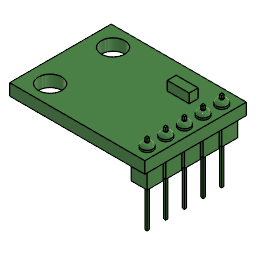
Dhanip_light-sensor (Autodesk Fusion 360 design; units mm, degrees)
Autodesk Fusion 360 part; units mm, degrees
note: some values were not read from the file. Set by a fixed rule: which sketch regions a step uses; which face or edge a step refers to.
sketch "Sketch1" plane through (0, 0, 0) normal (0, 0, 1) x (1, 0, 0)
sketch "Sketch2" plane through (0, 0, 0) normal (0, 0, 1) x (1, 0, 0)
  line L0 (9.25, -6.95) -> (-9.25, -6.95)
  line L1 (-9.25, -6.95) -> (-9.25, 6.95)
  line L2 (-9.25, 6.95) -> (9.25, 6.95)
  line L3 (9.25, 6.95) -> (9.25, -6.95)
  line L4 (9.25, -6.95) -> (-9.25, 6.95) construction
  line L5 (-9.25, -6.95) -> (9.25, 6.95) construction
  dimension "d3" = 18.5
  dimension "d4" = 13.9
  constraint horizontal L0
  constraint perpendicular L0 L1
  constraint parallel L0 L2
  constraint parallel L1 L3
  constraint coincident L4 origin
  constraint coincident L5 origin
  measures "d3" distance of L1.end L2.end
  measures "d4" distance of L0.end L1.end
extrude "Extrude1" add sketch "Sketch2" along normal blind 1.6
sketch "Sketch6" plane through (0, 0, 1.6) normal (0, 0, 1) x (-1, 0, 0)
  line L0 (-9.25, -6.95) -> (9.25, -6.95)
  line L1 (9.25, -6.95) -> (9.25, 6.95)
  line L2 (9.25, 6.95) -> (-9.25, 6.95)
  line L3 (-9.25, 6.95) -> (-9.25, -6.95)
  line L4 (9.25, 6.95) -> (6.35, 6.95)
  line L5 (9.25, 6.95) -> (9.25, 4.3)
  line L6 (9.25, 4.3) -> (5.4, 4.3)
  line L7 (6.35, 6.95) -> (6.35, 4.3)
  circle A0 centre (6.35, 4.3) radius 1.6
  dimension "d18" = 2.9
  dimension "d19" = 2.65
  dimension "d20" = 3.2
  constraint coincident L1.end L2.start
  constraint perpendicular L1 L4
  constraint perpendicular L2 L5
  constraint perpendicular L5 L6
  constraint coincident L6 L7.end
  constraint perpendicular L6 L7
  constraint coincident L7.end A0.centre
  measures "d18" distance of L1.end L4.end
  measures "d19" distance of L1.end L5.end
  measures "d20" diameter of A0
extrude "Extrude5" cut sketch "Sketch6" against normal blind 1.6 contours L6 L7 A0 | L6 L7 A0
mirror "Mirror2" about plane through (0, 0, 0) normal (0, 1, 0) of "Extrude5"
sketch "Sketch7" plane through (0, 0, 1.6) normal (0, 0, 1) x (-1, 0, 0)
  circle A0 centre (6.35, -4.3) radius 1.6
  circle A1 centre (6.35, 4.3) radius 1.6
  line L0 (-9.25, -6.95) -> (9.25, -6.95)
  line L1 (9.25, -6.95) -> (9.25, 6.95)
  line L2 (9.25, 6.95) -> (-9.25, 6.95)
  line L3 (-9.25, 6.95) -> (-9.25, -6.95)
  line L4 (-9.25, -4.9302) -> (-7.883, -4.9302)
  line L5 (-7.883, -4.9302) -> (-7.883, -6.95)
  line L6 (-7.883, -6.95) -> (-9.25, -6.95)
  line L7 (-7.883, -6.95) -> (-7.883, -4.926)
  circle A2 centre (-7.883, -4.9302) radius 0.7705
  dimension "d25" = 1.367
  dimension "d26" = 2.024
  dimension "d27" = 1.541
  constraint coincident L3 L4.start
  constraint perpendicular L3 L4
  constraint coincident L0 L5.end
  constraint perpendicular L0 L5
  constraint coincident L0.start L3.end
  constraint perpendicular L0 L7
  constraint coincident L4.end L5.start
  measures "d25" distance of L4.start L4.end
  measures "d26" distance of L5.end L7.end
  measures "d27" diameter of A2
extrude "Extrude6" add sketch "Sketch7" along normal blind 0.765 contours L4 L5 L7 A2 | L4 L5 L7 A2
sketch "Sketch8" plane through (0, 0, 2.365) normal (0, 0, 1) x (-1, 0, 0)
  circle A0 centre (-7.883, -4.9302) radius 0.7705
  line L0 (-7.733, -5.0802) -> (-8.033, -5.0802)
  line L1 (-8.033, -5.0802) -> (-8.033, -4.7802)
  line L2 (-8.033, -4.7802) -> (-7.733, -4.7802)
  line L3 (-7.733, -4.7802) -> (-7.733, -5.0802)
  line L4 (-7.733, -5.0802) -> (-8.033, -4.7802) construction
  line L5 (-8.033, -5.0802) -> (-7.733, -4.7802) construction
  point P0 (-7.883, -4.9302)
  dimension "d30" = 0.3
  dimension "d31" = 0.3
  constraint horizontal L0
  constraint perpendicular L0 L1
  constraint parallel L0 L2
  constraint parallel L1 L3
  constraint coincident L4 P0
  constraint coincident L5 P0
  constraint coincident P0 A0.centre
  measures "d30" distance of L1.end L2.end
  measures "d31" distance of L0.end L1.end
extrude "Extrude7" add sketch "Sketch8" along normal blind 0.531 contours L0 L1 L2 L3
fillet "Fillet1" radius 0.525 1 edges at (8.6014, 5.2088, 2.365)
pattern_linear "R-Pattern1" count 5 spacing 2.55 along (0, -1, 0) of "Extrude6", "Extrude7", "Fillet1"
extrude "Extrude8" add 5 faces at (7.833, 4.8802, 2.896) (7.833, 2.3302, 2.896) (7.833, -0.2198, 2.896) (7.833, -2.7698, 2.896) (7.833, -5.3198, 2.896) along direction (0, 0, -1) blind 11
sketch "Sketch9" plane through (0, 0, 0) normal (0, 0, -1) x (1, 0, 0)
  line L0 (8.033, 5.4198) -> (8.033, 5.1198)
  line L1 (8.033, 5.1198) -> (7.733, 5.1198)
  line L2 (7.733, 5.1198) -> (7.733, 5.4198)
  line L3 (7.733, 5.4198) -> (8.033, 5.4198)
  line L4 (8.033, 0.3198) -> (8.033, 0.0198)
  line L5 (8.033, 0.0198) -> (7.733, 0.0198)
  line L6 (7.733, 0.0198) -> (7.733, 0.3198)
  line L7 (7.733, 0.3198) -> (8.033, 0.3198)
  line L8 (8.033, -4.7802) -> (8.033, -5.0802)
  line L9 (8.033, -5.0802) -> (7.733, -5.0802)
  line L10 (7.733, -5.0802) -> (7.733, -4.7802)
  line L11 (7.733, -4.7802) -> (8.033, -4.7802)
  line L12 (8.033, -2.2302) -> (8.033, -2.5302)
  line L13 (8.033, -2.5302) -> (7.733, -2.5302)
  line L14 (7.733, -2.5302) -> (7.733, -2.2302)
  line L15 (7.733, -2.2302) -> (8.033, -2.2302)
  line L16 (8.033, 2.8698) -> (8.033, 2.5698)
  line L17 (8.033, 2.5698) -> (7.733, 2.5698)
  line L18 (7.733, 2.5698) -> (7.733, 2.8698)
  line L19 (7.733, 2.8698) -> (8.033, 2.8698)
  circle A0 centre (-6.35, -4.3) radius 1.6
  circle A1 centre (-6.35, 4.3) radius 1.6
  line L20 (-9.25, -6.95) -> (9.25, -6.95)
  line L21 (9.25, -6.95) -> (9.25, 6.95)
  line L22 (9.25, 6.95) -> (-9.25, 6.95)
  line L23 (-9.25, 6.95) -> (-9.25, -6.95)
  line L24 (7.733, 5.4198) -> (8.033, 5.1198)
  line L25 (7.733, 5.1198) -> (8.033, 5.4198)
  line L26 (8.983, 6.3698) -> (6.783, 6.3698)
  line L27 (6.783, 6.3698) -> (6.783, 4.1698)
  line L28 (6.783, 4.1698) -> (8.983, 4.1698)
  line L29 (8.983, 4.1698) -> (8.983, 6.3698)
  line L30 (8.983, 6.3698) -> (6.783, 4.1698) construction
  line L31 (6.783, 6.3698) -> (8.983, 4.1698) construction
  line L32 (7.733, 2.8698) -> (8.033, 2.5698)
  line L33 (8.033, 2.8698) -> (7.733, 2.5698)
  line L34 (8.983, 1.6198) -> (6.783, 1.6198)
  line L35 (6.783, 1.6198) -> (6.783, 3.8198)
  line L36 (6.783, 3.8198) -> (8.983, 3.8198)
  line L37 (8.983, 3.8198) -> (8.983, 1.6198)
  line L38 (8.983, 1.6198) -> (6.783, 3.8198) construction
  line L39 (6.783, 1.6198) -> (8.983, 3.8198) construction
  line L40 (7.733, 0.3198) -> (8.033, 0.0198)
  line L41 (7.733, 0.0198) -> (8.033, 0.3198)
  line L42 (8.983, -0.9302) -> (6.783, -0.9302)
  line L43 (6.783, -0.9302) -> (6.783, 1.2698)
  line L44 (6.783, 1.2698) -> (8.983, 1.2698)
  line L45 (8.983, 1.2698) -> (8.983, -0.9302)
  line L46 (8.983, -0.9302) -> (6.783, 1.2698) construction
  line L47 (6.783, -0.9302) -> (8.983, 1.2698) construction
  line L48 (7.733, -2.2302) -> (8.033, -2.5302)
  line L49 (7.733, -2.5302) -> (8.033, -2.2302)
  line L50 (7.733, -4.7802) -> (8.033, -5.0802)
  line L51 (7.733, -5.0802) -> (8.033, -4.7802)
  line L52 (8.983, -3.4802) -> (6.783, -3.4802)
  line L53 (6.783, -3.4802) -> (6.783, -1.2802)
  line L54 (6.783, -1.2802) -> (8.983, -1.2802)
  line L55 (8.983, -1.2802) -> (8.983, -3.4802)
  line L56 (8.983, -3.4802) -> (6.783, -1.2802) construction
  line L57 (6.783, -3.4802) -> (8.983, -1.2802) construction
  line L58 (8.983, -6.0302) -> (6.783, -6.0302)
  line L59 (6.783, -6.0302) -> (6.783, -3.8302)
  line L60 (6.783, -3.8302) -> (8.983, -3.8302)
  line L61 (8.983, -3.8302) -> (8.983, -6.0302)
  line L62 (8.983, -6.0302) -> (6.783, -3.8302) construction
  line L63 (6.783, -6.0302) -> (8.983, -3.8302) construction
  point P0 (7.883, 5.2698)
  point P1 (7.883, 2.7198)
  point P2 (7.883, 0.1698)
  point P3 (7.883, -2.3802)
  point P4 (7.883, -4.9302)
  dimension "d42" = 2.2
  dimension "d43" = 2.2
  dimension "d44" = 2.2
  dimension "d45" = 2.2
  dimension "d46" = 2.2
  dimension "d47" = 2.2
  dimension "d48" = 2.2
  dimension "d49" = 2.2
  dimension "d50" = 2.2
  dimension "d51" = 2.2
  constraint coincident L2.end L3.start
  constraint coincident L0.end L1.start
  constraint coincident L1.end L2.start
  constraint coincident L0.start L3.end
  constraint horizontal L26
  constraint perpendicular L26 L27
  constraint parallel L26 L28
  constraint parallel L27 L29
  constraint coincident L30 P0
  constraint coincident L31 P0
  constraint midpoint L25 P0
  constraint coincident L18.end L19.start
  constraint coincident L16.end L17.start
  constraint coincident L16.start L19.end
  constraint coincident L17.end L18.start
  constraint horizontal L34
  constraint perpendicular L34 L35
  constraint parallel L34 L36
  constraint parallel L35 L37
  constraint coincident L38 P1
  constraint coincident L39 P1
  constraint midpoint L33 P1
  constraint coincident L6.end L7.start
  constraint coincident L4.end L5.start
  constraint coincident L5.end L6.start
  constraint coincident L4.start L7.end
  constraint horizontal L42
  constraint perpendicular L42 L43
  constraint parallel L42 L44
  constraint parallel L43 L45
  constraint coincident L46 P2
  constraint coincident L47 P2
  constraint midpoint L40 P2
  constraint coincident L14.end L15.start
  constraint coincident L12.end L13.start
  constraint coincident L13.end L14.start
  constraint coincident L12.start L15.end
  constraint coincident L10.end L11.start
  constraint coincident L8.end L9.start
  constraint coincident L9.end L10.start
  constraint coincident L8.start L11.end
  constraint horizontal L52
  constraint perpendicular L52 L53
  constraint parallel L52 L54
  constraint parallel L53 L55
  constraint coincident L56 P3
  constraint coincident L57 P3
  constraint midpoint L49 P3
  constraint horizontal L58
  constraint perpendicular L58 L59
  constraint parallel L58 L60
  constraint parallel L59 L61
  constraint coincident L62 P4
  constraint coincident L63 P4
  constraint midpoint L50 P4
  measures "d42" distance of L27.end L28.end
  measures "d43" distance of L26.end L27.end
  measures "d44" distance of L35.end L36.end
  measures "d45" distance of L34.end L35.end
  measures "d46" distance of L43.end L44.end
  measures "d47" distance of L42.end L43.end
  measures "d48" distance of L53.end L54.end
  measures "d49" distance of L52.end L53.end
  measures "d50" distance of L59.end L60.end
  measures "d51" distance of L58.end L59.end
extrude "Extrude9" add sketch "Sketch9" along normal blind 2.309 contours L26 L27 L28 L29 | L34 L35 L36 L37 | L42 L43 L44 L45 | L52 L53 L54 L55 | L58 L59 L60 L61
sketch "Sketch10" plane through (0, 0, 1.6) normal (0, 0, 1) x (-1, 0, 0)
  circle A0 centre (-7.883, 5.2698) radius 0.7705
  circle A1 centre (-7.883, 2.7198) radius 0.7705
  circle A2 centre (-7.883, 0.1698) radius 0.7705
  circle A3 centre (-7.883, -2.3802) radius 0.7705
  circle A4 centre (-7.883, -4.9302) radius 0.7705
  circle A5 centre (6.35, -4.3) radius 1.6
  circle A6 centre (6.35, 4.3) radius 1.6
  line L0 (-9.25, -6.95) -> (9.25, -6.95)
  line L1 (9.25, -6.95) -> (9.25, 6.95)
  line L2 (9.25, 6.95) -> (-9.25, 6.95)
  line L3 (-9.25, 6.95) -> (-9.25, -6.95)
  line L4 (-9.25, -6.95) -> (-9.25, -3.37)
  line L5 (-9.25, -3.37) -> (-5.529, -3.37)
  line L6 (-5.5287, -2.8397) -> (-5.5287, -4.0597)
  line L7 (-5.5287, -4.0597) -> (-2.5287, -4.0597)
  line L8 (-2.5287, -4.0597) -> (-5.5287, -4.0597)
  line L9 (-5.5287, -4.0597) -> (-5.5287, -2.8397)
  line L10 (-5.5287, -2.8397) -> (-2.5287, -2.8397)
  line L11 (-2.5287, -2.8397) -> (-2.5287, -4.0597)
  dimension "d54" = 3.58
  dimension "d55" = 3.721
  dimension "d56" = 1.22
  dimension "d57" = 3
  constraint coincident L0.start L3.end
  constraint perpendicular L0 L4
  constraint perpendicular L3 L5
  constraint perpendicular L5 L6
  constraint perpendicular L6 L7
  constraint horizontal L8
  constraint vertical L9
  constraint horizontal L10
  constraint vertical L11
  measures "d54" distance of L0.start L4.end
  measures "d55" distance of L4.end L5.end
  measures "d56" distance of L6.start L6.end
  measures "d57" distance of L6.end L7.end
extrude "Extrude10" add sketch "Sketch10" along normal blind 1.261 contours L6 L7 L8 L9 L10 L11
extrude "Extrude11" cut 5 faces at (7.833, 4.8802, 2.896) (7.833, 2.3302, 2.896) (7.833, -0.2198, 2.896) (7.833, -2.7698, 2.896) (7.833, -5.3198, 2.896) along direction (0, 0, -1) blind 0.035
